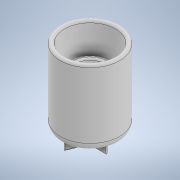
# Autodesk Inventor part: Potentiometer_Cap
Saved by Autodesk Inventor 2020 (Build 240168000, 168)
## iProperties
Created: 2020-05-25
Part Number: Potentiometer_Cap
Material: Generic
Document SubType Name: Modeling
Designer: maple
Density: 1 g/cm^3
Appearance: Default
Author: maple
Autodesk Inventor part; units mm, degrees
ref_plane "YZ Plane" through (0, 0, 0) normal (1, 0, 0) x (0, 1, 0)
ref_plane "XZ Plane" through (0, 0, 0) normal (0, 1, 0) x (-1, 0, 0)
ref_plane "XY Plane" through (0, 0, 0) normal (0, 0, 1) x (1, 0, 0)
sketch "Sketch1" plane through (0, 0, 0) normal (0, 1, 0) x (-1, 0, 0)
  circle A0 centre (0, 0) radius 7
  circle A1 centre (0, 0) radius 6
  circle A2 centre (0, 0) radius 3.5
  circle A3 centre (0, 0) radius 4.5
  line L0 (0, 0) -> (0.4, 0)
  line L1 (0, 0) -> (-0.4, 0)
  line L2 (-0.4, 0) -> (-0.4, -3.4771)
  line L3 (-0.4, 0) -> (-0.4, 3.4771)
  line L4 (0.4, 0) -> (0.4, -3.4771)
  line L5 (0.4, 0) -> (0.4, 3.4771)
  dimension "d0" = 14
  dimension "d1" = 12
  dimension "d2" = 7
  dimension "d3" = 9
  dimension "d4" = 0.4
  dimension "d5" = 0.4
  constraints: 12 end point, 4 centre point, 4 coincident, 4 point on circle, 2 horizontal, 2 point on line, 1 parallel, 1 perpendicular
  measures "d0" diameter of A0
  measures "d1" diameter of A1
  measures "d2" diameter of A2
  measures "d3" diameter of A3
  measures "d4" distance of L0.start L0.end
  measures "d5" distance of L0.start L1.end
sketch "Sketch2" plane through (0, 0, 0) normal (0, 1, 0) x (-1, 0, 0)
  circle A0 centre (0, 0) radius 7
  dimension "d6" = 14
  constraints: 1 centre point, 1 coincident
  measures "d6" diameter of A0
extrude "Extrusion1" add sketch "Sketch2" against normal blind 2
extrude "Extrusion2" add sketch "Sketch1" along normal blind 10 contours L5 L0 L1 L3 A2 | A2 L2 L1 L0 L4 | A3
sketch "Sketch3" plane through (0, 0, 0) normal (0, 1, 0) x (1, 0, 0)
  circle A0 centre (0, 0) radius 7
  circle A1 centre (0, 0) radius 6
  dimension "d11" = 14
  dimension "d12" = 12
  constraints: 2 centre point, 2 coincident
  measures "d11" diameter of A0
  measures "d12" diameter of A1
extrude "Extrusion3" add sketch "Sketch3" along normal blind 16
sketch "Sketch4" plane through (0, -2, 0) normal (0, -1, 0) x (1, 0, 0)
  line L0 (0, 0) -> (0, 6.5)
  line L1 (-6.1819, 2.0086) -> (6.1819, 2.0086)
  line L2 (6.1819, 2.0086) -> (-3.8206, -5.2586)
  line L3 (-3.8206, -5.2586) -> (0, 6.5)
  line L4 (3.8206, -5.2586) -> (0, 6.5)
  line L5 (-6.1819, 2.0086) -> (3.8206, -5.2586)
  point P0 (-2.3613, -0.7672)
  point P1 (0, -2.4828)
  point P2 (2.3613, -0.7672)
  point P3 (1.4593, 2.0086)
  point P4 (-1.4593, 2.0086)
  dimension "d15" = 6.5
  dimension "d18" = 360
  constraints: 12 end point, 1 horizontal, 1 vertical, 6 other
  measures "d15" distance of L0.start L0.end
extrude "Extrusion4" add sketch "Sketch4" along normal blind 2
chamfer "Chamfer1" distance 0.8 angle 45 10 edges at (-1.9103, -4, -3.8707) (-3.0909, -4, -3.0129) (1.9103, -4, -3.8707) (-4.2716, -4, 0.6207) (-3.8206, -4, 2.0086) (-0.7297, -4, 4.2543) (0.7297, -4, 4.2543) (3.8206, -4, 2.0086) (4.2716, -4, 0.6207) (3.0909, -4, -3.0129)
fillet "Fillet1" radius 2 1 edges at (7, -2, 0)
fillet "Fillet2" radius 0.2 5 edges at (0, -2.2614, 6.5) (6.1819, -2.2614, 2.0086) (3.8206, -2.2614, -5.2586) (-3.8206, -2.2614, -5.2586) (-6.1819, -2.2614, 2.0086)
fillet "Fillet4" radius 0.4 5 edges at (0.4, 10, 0) (-0.4, 10, 0) (3.5, 10, 0) (4.5, 10, 0) (-3.5, 10, 0)
fillet "Fillet5" radius 0.5 2 edges at (-6, 16, 0) (-7, 16, 0)
body "Solid1"
